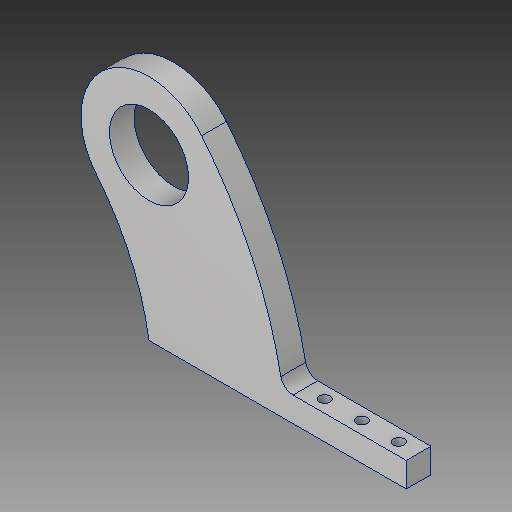
# Autodesk Inventor part: Idle Shooter holder
Saved by Autodesk Inventor 2019.4 (Build 234330000, 330)
## iProperties
Created: 2020-01-11
Part Number: Idle Shooter holder
Material: Aluminum 6061
Document SubType Name: Modeling
Designer: admin
Density: 2.7 g/cm^3
Appearance: Aluminum - Flat
Author: admin
Autodesk Inventor part; units mm, degrees
ref_plane "YZ Plane" through (0, 0, 0) normal (1, 0, 0) x (0, 1, 0)
ref_plane "XZ Plane" through (0, 0, 0) normal (0, 1, 0) x (-1, 0, 0)
ref_plane "XY Plane" through (0, 0, 0) normal (0, 0, 1) x (1, 0, 0)
sketch "Sketch1" plane through (0, 0, 0) normal (0, 0, 1) x (1, 0, 0)
  circle A0 centre (0, 0) radius 16
  arc A1 (-21.3037, -17.3897) -> (21.3037, 17.3897) centre (0, 0) ccw construction
  arc A2 (0, -65) -> (-21.3037, -17.3897) centre (-98.7718, -80.625) ccw
  arc A3 (54.0954, -55) -> (21.3037, 17.3897) centre (-98.7718, -80.625) ccw
  line L0 (54.0954, -55) -> (104.0954, -55)
  line L1 (104.0954, -55) -> (104.0954, -65)
  line L2 (104.0954, -65) -> (0, -65)
  arc A4 (21.3037, 17.3897) -> (-21.3037, -17.3897) centre (0, 0) ccw
  dimension "d0" = 32
  dimension "d1" = 55
  dimension "d2" = 10
  dimension "d3" = 65
  dimension "d4" = 100
  dimension "d5" = 50
  dimension "d6" = 0
  constraints: 8 point on circle, 6 end point, 5 centre point, 3 coincident, 2 perpendicular, 2 tangent, 1 horizontal
  measures "d0" diameter of A0
  measures "d1" diameter of A1
  measures "d2" distance of L0.end L1.end
  measures "d3" distance from line of point (0, 0) L2
  measures "d4" radius of A2
  measures "d5" distance of L0.start L0.end
  measures "d6" horizontal distance of L2.end point (0, 0)
extrude "Extrusion1" add sketch "Sketch1" along normal blind 10
fillet "Fillet1" radius 5 1 edges at (54.0954, -55, 5)
sketch "Sketch2" plane through (104.0954, -55, 10) normal (0, 1, 0) x (1, 0, 0)
  circle A0 centre (-38, 5) radius 2.2
  circle A1 centre (-23, 5) radius 2.2
  circle A2 centre (-8, 5) radius 2.2
  line L0 (-8, 5) -> (-38, 5) construction
  line L1 (0, 10) -> (0, 0) projected
  line L2 (0, 10) -> (-45.8254, 10) projected
  point P0 (-104.0954, 10)
  dimension "d10" = 4.4
  dimension "d11" = 4.4
  dimension "d12" = 4.4
  dimension "d13" = 30
  dimension "d14" = 8
  dimension "d15" = 5
  constraints: 3 centre point, 2 end point, 1 coincident, 1 horizontal, 1 midpoint
  measures "d10" diameter of A0
  measures "d11" diameter of A1
  measures "d12" diameter of A2
  measures "d13" distance of L0.start L0.end
  measures "d14" distance from line of L1 L0.start
  measures "d15" distance between parallel lines of L2 L0
extrude "Extrusion2" cut sketch "Sketch2" against normal through all
body "Solid1"
